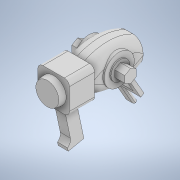
# Autodesk Inventor part: Weapon-Healing-Body
Saved by Autodesk Inventor 2020 (Build 240168000, 168)
## iProperties
Created: 2019-12-02
Part Number: Weapon-Healing-Body
Material: Generic
Document SubType Name: Modeling
Designer: vifly_01
Density: 1 g/cm^3
Appearance: Default
Author: vifly_01
Autodesk Inventor part; units mm, degrees
ref_plane "YZ Plane" through (0, 0, 0) normal (1, 0, 0) x (0, 1, 0)
ref_plane "XZ Plane" through (0, 0, 0) normal (0, 1, 0) x (-1, 0, 0)
ref_plane "XY Plane" through (0, 0, 0) normal (0, 0, 1) x (1, 0, 0)
sketch "Sketch1" plane through (0, 0, 0) normal (0, 0, 1) x (1, 0, 0)
  circle A0 centre (0, 0) radius 5
  dimension "d0" = 10
  constraints: 1 centre point, 1 coincident
  measures "d0" diameter of A0
extrude "Extrusion1" add sketch "Sketch1" along normal blind 2.5 draft -10
sketch "Sketch2" plane through (0, 0, 0) normal (0, 0, -1) x (-1, 0, 0)
  line L0 (-6.25, -6.25) -> (6.25, -6.25)
  line L1 (6.25, -6.25) -> (6.25, 6.25)
  line L2 (6.25, 6.25) -> (-6.25, 6.25)
  line L3 (-6.25, 6.25) -> (-6.25, -6.25)
  line L4 (-6.25, -6.25) -> (6.25, 6.25) construction
  line L5 (6.25, -6.25) -> (-6.25, 6.25) construction
  point P0 (0, 0)
  dimension "d3" = 12.5
  dimension "d4" = 12.5
  constraints: 12 end point, 2 midpoint, 2 parallel, 1 horizontal, 1 perpendicular
  measures "d3" distance of L2.end L1.end
  measures "d4" distance of L1.end L0.end
extrude "Extrusion2" add sketch "Sketch2" along normal blind 10
sketch "Sketch3" plane through (0, 0, 0) normal (1, 0, 0) x (0, 1, 0)
  line L0 (7.5, -10) -> (7.5, -30)
  line L1 (7.5, -30) -> (-7.5, -30)
  line L2 (-7.5, -30) -> (-7.5, -10)
  line L3 (-7.5, -10) -> (7.5, -10)
  point P0 (0, 0)
  dimension "d7" = 20
  dimension "d8" = 15
  constraints: 8 end point, 2 parallel, 1 perpendicular, 1 vertical
  measures "d7" distance of L0.start L0.end
  measures "d8" distance of L0.end L1.end
extrude "Extrusion3" add sketch "Sketch3" along normal mid plane 11
sketch "Sketch4" plane through (0, 0, 0) normal (1, 0, 0) x (0, 1, 0)
  line L0 (7.5, -30) -> (-7.5, -30) projected
  line L1 (-6.25, -10) -> (6.25, -10) projected
  line L2 (7.5, -30) -> (7.5, -10) projected
  line L3 (-6.25, -10) -> (6.25, -10) projected
  arc A0 (5, -30) -> (5, -10) centre (-13.75, -20) ccw
  line L4 (5, -10) -> (5, -30) construction
  line L5 (5, -10) -> (25, -10) construction
  arc A1 (-5, -10) -> (-5, -30) centre (13.75, -20) ccw
  line L6 (-5, -10) -> (-5, -30) construction
  line L7 (-5, -10) -> (15, -10) construction
  line L8 (6.25, -10) -> (7.5, -10) projected
  line L9 (5, -10) -> (7.5, -10)
  line L10 (7.5, -10) -> (7.5, -20)
  line L11 (7.5, -10) -> (7.5, -30) projected
  line L12 (7.5, -20) -> (7.5, -30)
  line L13 (7.5, -30) -> (5, -30)
  line L14 (-7.5, -30) -> (-7.5, -10) projected
  line L15 (-5, -30) -> (-7.5, -30)
  line L16 (-7.5, -30) -> (-7.5, -20)
  line L17 (-7.5, -10) -> (-6.25, -10) projected
  line L18 (-7.5, -20) -> (-7.5, -10)
  line L19 (-7.5, -10) -> (-5, -10)
  point P0 (0, 0)
  point P1 (-7.5, -20)
  point P2 (-5, -10)
  point P3 (5, -10)
  point P4 (7.5, -20)
  dimension "d11" = 90
  dimension "d12" = 90
  dimension "d58" = 2.5
  constraints: 24 end point, 5 point on circle, 4 point on line, 3 collinear, 3 horizontal, 2 centre point, 2 perpendicular, 2 vertical, 1 midpoint
  measures "d11" angle of L4 L5
  measures "d12" angle of L6 L7
  measures "d58" horizontal distance of L4.start L10.end
extrude "Extrusion4" cut sketch "Sketch4" along normal mid plane 11 contours L0 A0 L2 | A0 L1 L8 L2 | L0 L14 A1 | L14 L17 L1 A1
fillet "Fillet1" radius 2 4 edges at (6.25, 6.25, -5) (6.25, -6.25, -5) (-6.25, 6.25, -5) (-6.25, -6.25, -5)
fillet "Fillet2" radius 4 4 edges at (5.5, 7.5, -20) (5.5, -7.5, -20) (-5.5, -7.5, -20) (-5.5, 7.5, -20)
sketch "Sketch5" plane through (5.5, 0, 0) normal (1, 0, 0) x (0, 0, -1)
  circle A0 centre (20, 0) radius 6
  point P0 (0, 0)
  dimension "d17" = 12
  constraints: 1 centre point
  measures "d17" diameter of A0
extrude "Extrusion5" add sketch "Sketch5" against normal blind 0.9
sketch "Sketch6" plane through (5.5, 0, 0) normal (1, 0, 0) x (0, 0, -1)
  circle A0 centre (20, 0) radius 6
  point P0 (0, 0)
  constraints: 1 centre point
extrude "Extrusion6" add sketch "Sketch6" along normal blind 0.5
sketch "Sketch9" plane through (6, 0, -20) normal (1, 0, 0) x (0, 0, -1)
  circle A0 centre (0, 0) radius 3.75
  point P0 (-20, 0)
  dimension "d26" = 7.5
  constraints: 1 centre point
  measures "d26" diameter of A0
extrude "Extrusion9" add sketch "Sketch9" along normal blind 0.5
sketch "Sketch10" plane through (6.5, 0, -20) normal (1, 0, 0) x (0, 0, -1)
  line L0 (0.0215, 2.6293) -> (2.2986, 1.3147)
  line L1 (2.2986, 1.3147) -> (2.2986, -1.3147)
  line L2 (2.2986, -1.3147) -> (0.0215, -2.6293)
  line L3 (0.0215, -2.6293) -> (-2.2556, -1.3147)
  line L4 (-2.2556, -1.3147) -> (-2.2556, 1.3147)
  line L5 (-2.2556, 1.3147) -> (0.0215, 2.6293)
  point P0 (-20, 0)
  point P1 (0.0215, 0)
  constraints: 12 end point, 1 vertical alignment, 13 other
extrude "Extrusion10" add sketch "Sketch10" along normal blind 4
mirror "Mirror1" about plane through (0, 0, 0) normal (1, 0, 0) of "Extrusion5", "Extrusion6", "Extrusion9", "Extrusion10"
sketch "Sketch11" plane through (0, 0, 0) normal (1, 0, 0) x (0, 1, 0)
  line L0 (-6.25, -10) -> (-6.25, 0) projected
  line L1 (-6.25, -6.9595) -> (-20.6651, -10)
  line L2 (-20.6651, -10) -> (-21.9685, -3.8204)
  line L3 (-21.9685, -3.8204) -> (-20.6651, -3.5455)
  line L4 (-7.2105, -2.4056) -> (-6.25, -2.203)
  line L5 (-7.2105, -2.4056) -> (-17.8743, -4.6548)
  arc A0 (-20.6651, -3.5455) -> (-17.8743, -4.6548) centre (-18.4345, -1.9988) ccw
  line L6 (-6.25, -2.203) -> (-6.25, -6.9595)
  point P0 (0, 0)
  dimension "d31" = 6.1796
  constraints: 12 end point, 2 perpendicular, 2 point on circle, 2 point on line, 1 centre point, 1 collinear, 1 tangent
  measures "d31" vertical distance of L1.end L2.end
extrude "Extrusion11" add sketch "Sketch11" along normal mid plane 4
ref_plane "Work Plane1" through (8.5, 2.6293, -20.0215) normal (1, 0, 0) x (0, 0, -1)
sketch "Sketch15" plane through (8.5, 2.6293, -20.0215) normal (1, 0, 0) x (0, 0, -1)
  line L0 (2.2771, -3.944) -> (0, -5.2587) projected
  line L1 (1.7881, -4.2263) -> (6.3593, -12.144)
  line L2 (0.489, -4.9763) -> (5.0603, -12.894)
  line L3 (5.0603, -12.894) -> (6.3593, -12.144)
  line L4 (0.489, -4.9763) -> (1.7881, -4.2263)
  point P0 (-20.0215, -2.6293)
  point P1 (1.7881, -4.2263)
  point P2 (0.489, -4.9763)
  dimension "d36" = 1.5
  dimension "d37" = 90
  dimension "d38" = 9.1425
  dimension "d39" = 7.9177
  dimension "d40" = 7.9177
  dimension "d41" = 1.299
  dimension "d42" = 16.5891
  constraints: 8 end point
  measures "d36" distance between parallel lines of L2 L1
  measures "d37" angle of L1 L0
  measures "d38" distance from line of L2.end L0
  measures "d39" vertical distance of L1.start L1.end
  measures "d40" vertical distance of L2.start L2.end
  measures "d41" horizontal distance of L2.end L1.end
  measures "d42" distance from line of L2 point (-20.022, -2.629)
extrude "Extrusion12" add sketch "Sketch15" along normal mid plane 2
ref_plane "Work Plane2" through (9.5, -1.972, -21.16) normal (0, 0.5, -0.8660254) x (-1, 0, 0)
sketch "Sketch16" plane through (9.5, -1.972, -21.16) normal (0, 0.5, -0.8660254) x (-1, 0, 0)
  line L0 (2, -9.1425) -> (0, -9.1425) projected
  line L1 (9.5, -7.1425) -> (0, -7.1425)
  line L2 (0, -7.1425) -> (0, -9.1425)
  line L3 (9.5, -19.1425) -> (7.5, -19.1425)
  line L4 (7.5, -19.1425) -> (7.5, -9.1425)
  line L5 (7.5, -9.1425) -> (9.5, -9.1425)
  line L6 (0, -9.1425) -> (7.5, -9.1425)
  line L7 (9.5, -7.1425) -> (9.5, -19.1425)
  point P0 (9.5, 12.2878)
  point P1 (2, -9.1425)
  dimension "d47" = 10
  dimension "d49" = 2
  dimension "d50" = 2
  dimension "d53" = 90
  constraints: 14 end point, 2 parallel, 1 horizontal, 1 perpendicular
  measures "d47" distance of L5.end L3.start
  measures "d49" distance of L3.start L3.end
  measures "d50" distance from line of L5.end L4
  measures "d53" angle of L3 L4
extrude "Extrusion13" add sketch "Sketch16" along normal mid plane 1.5
mirror "Mirror2" about plane through (0, 0, 0) normal (1, 0, 0) of "Extrusion13", "Extrusion12"
fillet "Fillet3" radius 1 4 edges at (2, -13.8448, -28.8808) (2, -14.5948, -27.5818) (-2, -13.8448, -28.8808) (-2, -14.5948, -27.5818)
equation "\"d4\" = d3"
body "Solid1"
